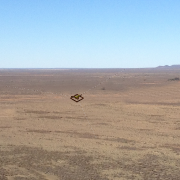
# Autodesk Inventor part: hub_jig
Saved by Autodesk Inventor 2013 (Build 170138000, 138)
## iProperties
Created: 2013-06-07
Part Number: hub_jig
Material: Wood (Walnut)
Document SubType Name: Modeling
Designer: David DeBoer
Density: 0.55 g/cm^3
Description: Hub jig for outer sonotube
Mass: 23487.8 g
Surface Area: 19224.8 cm^2
Volume: 42705 cm^3
Author: David DeBoer
Autodesk Inventor part; units mm, degrees
ref_plane "YZ Plane" through (0, 0, 0) normal (1, 0, 0) x (0, 1, 0)
ref_plane "XZ Plane" through (0, 0, 0) normal (0, 1, 0) x (-1, 0, 0)
ref_plane "XY Plane" through (0, 0, 0) normal (0, 0, 1) x (1, 0, 0)
sketch "Sketch1" plane through (0, 0, 0) normal (0, 1, 0) x (-1, 0, 0)
  line L0 (0, 0) -> (914.4, 0)
  line L1 (914.4, 0) -> (914.4, 914.4)
  line L2 (914.4, 914.4) -> (0, 914.4)
  line L3 (0, 914.4) -> (0, 0)
  line L4 (-50, 964.4) -> (964.4, 964.4)
  line L5 (964.4, 964.4) -> (964.4, -50)
  line L6 (964.4, -50) -> (-50, -50)
  line L7 (-50, -50) -> (-50, 964.4)
  dimension "d0" = 914.4
  dimension "d1" = 914.4
  dimension "d2" = 50
  constraints: 16 end point, 4 parallel, 2 perpendicular, 1 horizontal, 3 other
  measures "d0" distance of L0.start L0.end
  measures "d1" distance of L2.end L0.start
  measures "d2" distance between parallel lines of L2 L4
extrude "Extrusion1" add sketch "Sketch1" along normal blind 100
chamfer "Chamfer1" distance 101.6 angle 45 4 edges at (-914.4, 50, 914.4) (-914.4, 50, 0) (0, 50, 914.4) (0, 50, 0)
sketch "Sketch10" plane through (0, 100, 0) normal (0, 1, 0) x (1, 0, 0)
  line L0 (-964.4, -964.4) -> (50, -964.4) projected
  line L1 (50, -964.4) -> (50, 50) projected
  line L2 (50, 50) -> (-964.4, 50) projected
  line L3 (-457.2, 50) -> (-457.2, -964.4) construction
  line L4 (-457.2, -457.2) -> (50, -750.0321) construction
  line L5 (-457.2, -457.2) -> (128.4641, -457.2) construction
  line L6 (-457.2, -457.2) -> (-964.4, -750.0321) construction
  line L7 (-482.2698, 203.3987) -> (-482.2698, -457.0013)
  line L8 (-431.4698, 203.3987) -> (-431.4698, -457.0013)
  line L9 (-482.2698, 203.3987) -> (-431.4698, 203.3987)
  line L10 (-482.2698, -457.0013) -> (-431.4698, -457.0013)
  point P0 (0, 0)
  dimension "d32" = 30
  dimension "d33" = 25.0698
  dimension "d50" = 660.4
  constraints: 16 end point, 3 midpoint, 2 perpendicular, 1 equal length, 1 horizontal, 1 parallel, 1 point on line, 1 symmetric about line
  measures "d32" angle of L4 L5
  measures "d33" distance between parallel lines of L3 L7
  measures "d50" distance of L7.start L7.end
extrude "Extrusion7" add sketch "Sketch10" along normal blind 101.6
sketch "Sketch11" plane through (0, 201.6, 0) normal (0, 1, 0) x (1, 0, 0)
  line L0 (-462.4808, -319.9213) -> (-449.7808, -319.9213)
  line L1 (-449.7808, -319.9213) -> (-449.7808, 7300.0787)
  line L2 (-449.7808, 7300.0787) -> (-462.4808, 7300.0787)
  line L3 (-462.4808, 7300.0787) -> (-462.4808, -319.9213)
  point P0 (0, 0)
  dimension "d37" = 12.7
  dimension "d39" = 7620
  constraints: 8 end point, 2 parallel, 1 horizontal, 1 perpendicular
  measures "d37" distance of L0.start L0.end
  measures "d39" distance of L2.end L0.start
extrude "Extrusion8" add sketch "Sketch11" along normal blind 2.54
sketch "Sketch12" plane through (0, 100, 0) normal (0, -1, 0) x (1, 0, 0)
  line L0 (-482.2698, 457.0013) -> (-431.4698, 457.0013) projected
  circle A0 centre (-456.8698, 457.0013) radius 222.25
  point P0 (0, 0)
  dimension "d42" = 444.5
  constraints: 1 centre point, 1 midpoint
  measures "d42" diameter of A0
extrude "Extrusion9" add sketch "Sketch12" along normal blind 25.4
pattern_circular "Circular Pattern1" count 3 over 360 about axis through (-456.8698, 100, 457.0013) along (0, -1, 0) of "Extrusion7", "Extrusion8"
sketch "Sketch13" plane through (0, 201.6, 0) normal (0, 1, 0) x (1, 0, 0)
  line L0 (-466.0028, -71.0768) -> (-446.9528, -71.0768)
  line L1 (-446.9528, -71.0768) -> (-446.9528, -528.2768)
  line L2 (-446.9528, -528.2768) -> (-466.0028, -528.2768)
  line L3 (-466.0028, -528.2768) -> (-466.0028, -71.0768)
  line L4 (-684.633, -570.8547) -> (-684.633, -551.8047)
  line L5 (-684.633, -551.8047) -> (-227.433, -551.8047)
  line L6 (-227.433, -551.8047) -> (-227.433, -570.8547)
  line L7 (-227.433, -570.8547) -> (-684.633, -570.8547)
  point P0 (0, 0)
  dimension "d51" = 457.2
  dimension "d53" = 19.05
  dimension "d54" = 457.2
  dimension "d55" = 19.05
  constraints: 16 end point, 4 parallel, 2 perpendicular, 1 horizontal
  measures "d51" distance of L2.end L0.start
  measures "d53" distance of L1.end L2.end
  measures "d54" distance of L7.start L7.end
  measures "d55" distance of L5.end L7.start
extrude "Extrusion10" add sketch "Sketch13" along normal blind 76.2
sketch "Sketch14" plane through (-603.2696, 201.6, 570.8547) normal (0, 0, 1) x (1, 0, 0)
  line L0 (-81.3634, 76.2) -> (375.8366, 76.2) projected
  line L1 (-30.5634, 19.05) -> (45.6366, 19.05)
  line L2 (58.3366, 31.75) -> (58.3366, 44.45)
  line L3 (45.6366, 57.15) -> (-30.5634, 57.15)
  line L4 (-43.2634, 44.45) -> (-43.2634, 31.75)
  line L5 (147.2366, 76.2) -> (147.2366, 39.9206) construction
  arc A0 (-30.5634, 57.15) -> (-43.2634, 44.45) centre (-30.5634, 44.45) ccw
  arc A1 (58.3366, 44.45) -> (45.6366, 57.15) centre (45.6366, 44.45) ccw
  arc A2 (45.6366, 19.05) -> (58.3366, 31.75) centre (45.6366, 31.75) ccw
  arc A3 (-43.2634, 31.75) -> (-30.5634, 19.05) centre (-30.5634, 31.75) ccw
  line L6 (325.0366, 19.05) -> (248.8366, 19.05)
  line L7 (236.1366, 31.75) -> (236.1366, 44.45)
  line L8 (248.8366, 57.15) -> (325.0366, 57.15)
  line L9 (337.7366, 44.45) -> (337.7366, 31.75)
  arc A4 (337.7366, 44.45) -> (325.0366, 57.15) centre (325.0366, 44.45) ccw
  arc A5 (248.8366, 57.15) -> (236.1366, 44.45) centre (248.8366, 44.45) ccw
  arc A6 (236.1366, 31.75) -> (248.8366, 19.05) centre (248.8366, 31.75) ccw
  arc A7 (325.0366, 19.05) -> (337.7366, 31.75) centre (325.0366, 31.75) ccw
  line L10 (92.267, 30.0937) -> (92.267, 42.004)
  arc A8 (92.267, 30.0937) -> (104.967, 17.3937) centre (104.967, 30.0937) ccw
  arc A9 (104.967, 54.704) -> (92.267, 42.004) centre (104.967, 42.004) ccw
  line L11 (188.5218, 17.3937) -> (104.967, 17.3937)
  line L12 (104.967, 54.704) -> (188.5218, 54.704)
  line L13 (201.2218, 42.004) -> (201.2218, 30.0937)
  arc A10 (201.2218, 42.004) -> (188.5218, 54.704) centre (188.5218, 42.004) ccw
  arc A11 (188.5218, 17.3937) -> (201.2218, 30.0937) centre (188.5218, 30.0937) ccw
  line L14 (-81.3634, 0) -> (-81.3634, 76.2) projected
  point P0 (603.2696, -201.6)
  dimension "d58" = 12.7
  dimension "d64" = 76.2
  dimension "d65" = 12.7
  dimension "d66" = 38.1
  dimension "d71" = 19.05
  constraints: 26 end point, 24 point on circle, 12 centre point, 12 symmetric about line, 8 tangent, 3 equal radius, 3 parallel, 1 horizontal, 1 midpoint, 1 perpendicular, 4 other
  measures "d58" radius of A0
  measures "d64" distance of L1.start L1.end
  measures "d65" distance of L4.start L4.end
  measures "d66" distance between parallel lines of L4 L14
  measures "d71" distance between parallel lines of L3 L0
extrude "Extrusion11" cut sketch "Sketch14" against normal blind 25.4
sketch "Sketch15" plane through (-446.9528, 201.6, 528.2768) normal (1, 0, 0) x (0, 0, -1)
  line L0 (0, 76.2) -> (457.2, 76.2) projected
  line L1 (0, 0) -> (0, 76.2) projected
  line L2 (36.2205, 0) -> (0, 0) projected
  line L3 (228.6, 76.2) -> (228.6, 43.3162) construction
  line L4 (50.8, 19.05) -> (127, 19.05)
  line L5 (139.7, 31.75) -> (139.7, 44.45)
  line L6 (127, 57.15) -> (50.8, 57.15)
  line L7 (38.1, 44.45) -> (38.1, 31.75)
  arc A0 (50.8, 57.15) -> (38.1, 44.45) centre (50.8, 44.45) ccw
  arc A1 (139.7, 44.45) -> (127, 57.15) centre (127, 44.45) ccw
  arc A2 (127, 19.05) -> (139.7, 31.75) centre (127, 31.75) ccw
  arc A3 (38.1, 31.75) -> (50.8, 19.05) centre (50.8, 31.75) ccw
  line L8 (406.4, 19.05) -> (330.2, 19.05)
  line L9 (317.5, 31.75) -> (317.5, 44.45)
  line L10 (330.2, 57.15) -> (406.4, 57.15)
  line L11 (419.1, 44.45) -> (419.1, 31.75)
  arc A4 (419.1, 44.45) -> (406.4, 57.15) centre (406.4, 44.45) ccw
  arc A5 (330.2, 57.15) -> (317.5, 44.45) centre (330.2, 44.45) ccw
  arc A6 (317.5, 31.75) -> (330.2, 19.05) centre (330.2, 31.75) ccw
  arc A7 (406.4, 19.05) -> (419.1, 31.75) centre (406.4, 31.75) ccw
  line L12 (177.4731, 31.75) -> (177.4731, 44.45)
  arc A8 (190.1731, 57.15) -> (177.4731, 44.45) centre (190.1731, 44.45) ccw
  line L13 (266.3731, 19.05) -> (190.1731, 19.05)
  line L14 (190.1731, 57.15) -> (266.3731, 57.15)
  line L15 (279.0731, 44.45) -> (279.0731, 31.75)
  arc A9 (279.0731, 44.45) -> (266.3731, 57.15) centre (266.3731, 44.45) ccw
  arc A10 (266.3731, 19.05) -> (279.0731, 31.75) centre (266.3731, 31.75) ccw
  arc A11 (177.4731, 31.75) -> (190.1731, 19.05) centre (190.1731, 31.75) ccw
  point P0 (528.2768, -201.6)
  dimension "d61" = 12.7
  dimension "d62" = 76.2
  dimension "d63" = 12.7
  dimension "d67" = 38.1
  dimension "d68" = 19.05
  constraints: 26 end point, 24 point on circle, 12 centre point, 12 symmetric about line, 8 tangent, 3 equal radius, 2 parallel, 2 perpendicular, 1 horizontal, 1 midpoint, 4 other
  measures "d61" radius of A0
  measures "d62" distance of L4.start L4.end
  measures "d63" distance of L5.start L5.end
  measures "d67" distance between parallel lines of L7 L1
  measures "d68" distance between parallel lines of L6 L0
extrude "Extrusion12" cut sketch "Sketch15" against normal blind 25.4
sketch "Sketch16" plane through (-914.4, 100, 691.8271) normal (0, -1, 0) x (1, 0, 0)
  line L0 (253.6172, -146.4259) -> (0, 0) projected
  arc A0 (279.0172, -102.4318) -> (253.6172, -146.4259) centre (457.5302, -234.8258) ccw projected
  line L1 (0, 58.6588) -> (279.0172, -102.4318) projected
  circle A1 centre (457.5302, -234.8258) radius 444.5 construction
  line L2 (85.9109, 9.0581) -> (60.5109, -34.936)
  line L3 (107.908, -3.6419) -> (82.508, -47.636)
  line L4 (85.9109, 9.0581) -> (107.908, -3.6419)
  line L5 (60.5109, -34.936) -> (82.508, -47.636)
  point P0 (914.4, -691.8271)
  dimension "d72" = 889
  dimension "d73" = 25.4
  constraints: 8 end point, 2 perpendicular, 2 point on circle, 2 point on line, 1 centre point, 1 coincident, 1 parallel
  measures "d72" diameter of A1
  measures "d73" distance between parallel lines of L3 L2
extrude "Extrusion13" add sketch "Sketch16" along normal blind 50.8 contours L0 L2 L1 L3
pattern_circular "Circular Pattern2" count 3 over 360 about axis through (-456.8698, 100, 457.0013) along (0, -1, 0) of "Extrusion13"
body "Solid1"
